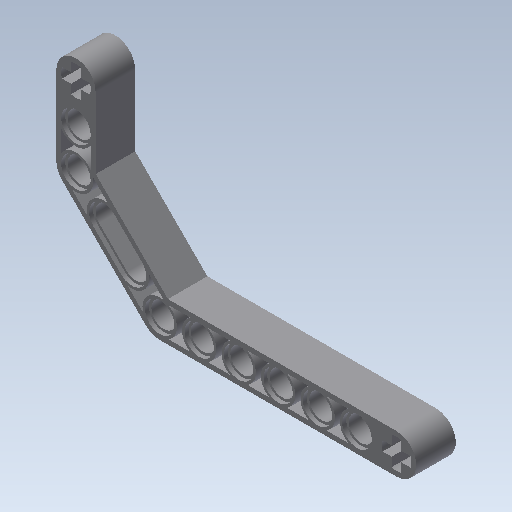
# Autodesk Inventor part: Arm Beam
Saved by Autodesk Inventor 2020 (Build 240168000, 168)
## iProperties
Created: 2014-02-19
Part Number: Arm Beam
Document SubType Name: Modeling
Designer: jleonard
Density: 1 g/cm^3
Material: Generic
Appearance: Default
Author: jleonard
Autodesk Inventor part; units mm, degrees
ref_plane "YZ Plane" through (0, 0, 0) normal (1, 0, 0) x (0, 1, 0)
ref_plane "XZ Plane" through (0, 0, 0) normal (0, 1, 0) x (-1, 0, 0)
ref_plane "XY Plane" through (0, 0, 0) normal (0, 0, 1) x (1, 0, 0)
sketch "Sketch1" plane through (0, 0, 0) normal (0, 0, 1) x (1, 0, 0)
  arc A0 (24, -4) -> (24, 4) centre (24, 0) ccw
  arc A1 (-44.9706, 16.9706) -> (-43.799, 14.1421) centre (-40.9706, 16.9706) ccw
  arc A2 (-36.9706, 32.9706) -> (-44.9706, 32.9706) centre (-40.9706, 32.9706) ccw
  line L0 (24, 4) -> (-22.3431, 4)
  line L1 (-22.3431, 4) -> (-36.9706, 18.6274)
  line L2 (-36.9706, 18.6274) -> (-36.9706, 32.9706)
  line L3 (24, -4) -> (-24, -4)
  line L4 (-26.8284, -2.8284) -> (-43.799, 14.1421)
  line L5 (-44.9706, 16.9706) -> (-44.9706, 32.9706)
  arc A3 (-26.8284, -2.8284) -> (-24, -4) centre (-24, 0) ccw
  line L6 (-59.9022, 0) -> (42.6504, 0) projected
  line L7 (0, -12.5317) -> (0, 45.2209) projected
  point P0 (0, 0)
  dimension "d4" = 48
  dimension "d6" = 16
  dimension "d9" = 24
  dimension "d12" = 4
  dimension "d13" = 4
  dimension "d14" = 4
  dimension "d15" = 4
  dimension "d16" = 135
  dimension "d17" = 135
  dimension "d18" = 4
  dimension "d19" = 4
  dimension "d20" = 4
  dimension "d21" = 4
  dimension "d22" = 24
  dimension "d23" = 0
  dimension "d25" = 4
  dimension "d26" = 4
  dimension "d27" = 8
  dimension "d28" = 8
  dimension "d29" = 22.3432
  dimension "d30" = 36.9706
  constraints: 12 end point, 8 point on circle, 4 centre point, 2 perpendicular
  measures "d4" distance of A3.centre A0.centre
  measures "d6" distance of A1.centre A2.centre
  measures "d9" distance of A3.centre A1.centre
  measures "d12" radius of A2
  measures "d13" radius of A1
  measures "d14" radius of A3
  measures "d15" radius of A0
  measures "d16" angle of L0 L1
  measures "d17" angle of L4 L3
  measures "d18" distance from line of L3 A0.centre
  measures "d19" distance from line of L2 A2.centre
  measures "d20" distance from line of L4 A1.centre
  measures "d21" distance from line of L1 A3.centre
  measures "d22" distance from line of A0.centre L7
  measures "d23" distance from line of A0.centre L6
  measures "d25" distance from line of L1 A1.centre
  measures "d26" distance from line of L0 A3.centre
  measures "d27" distance between parallel lines of L5 L2
  measures "d28" distance between parallel lines of L3 L0
  measures "d29" distance from line of L7 L0.end
  measures "d30" distance from line of L7 L1.end
extrude "Extrusion1" add sketch "Sketch1" along normal blind 8
sketch "Sketch2" plane through (0, 0, 8) normal (0, 0, 1) x (1, 0, 0)
  arc A0 (24, -4) -> (24, 4) centre (24, 0) ccw projected
  line L0 (24, -4) -> (-24, -4) projected
  arc A1 (21.1716, 1) -> (21.1716, -1) centre (24, 0) ccw
  arc A2 (23, -2.8284) -> (25, -2.8284) centre (24, 0) ccw
  arc A3 (26.8284, -1) -> (26.8284, 1) centre (24, 0) ccw
  arc A4 (25, 2.8284) -> (23, 2.8284) centre (24, 0) ccw
  line L1 (21.1716, 1) -> (23, 1)
  line L2 (25, 1) -> (26.8284, 1)
  line L3 (23, -2.8284) -> (23, -1)
  line L4 (23, 1) -> (23, 2.8284)
  line L5 (21.1716, -1) -> (23, -1)
  line L6 (25, -1) -> (26.8284, -1)
  line L7 (25, 2.8284) -> (25, 1)
  line L8 (25, -1) -> (25, -2.8284)
  point P0 (0, 0)
  dimension "d34" = 3
  dimension "d35" = 3
  dimension "d36" = 3
  dimension "d37" = 3
  dimension "d38" = 2
  dimension "d39" = 2
  dimension "d40" = 2
  dimension "d41" = 2
  dimension "d42" = 1
  dimension "d43" = 1
  dimension "d44" = 1
  dimension "d45" = 1
  constraints: 16 end point, 8 parallel, 8 point on circle, 6 perpendicular, 4 centre point, 1 coincident
  measures "d34" radius of A4
  measures "d35" radius of A3
  measures "d36" radius of A2
  measures "d37" radius of A1
  measures "d38" distance between parallel lines of L7 L4
  measures "d39" distance between parallel lines of L5 L1
  measures "d40" distance between parallel lines of L6 L2
  measures "d41" distance between parallel lines of L8 L3
  measures "d42" distance from line of A0.centre L4
  measures "d43" distance from line of A0.centre L1
  measures "d44" distance from line of A0.centre L3
  measures "d45" distance from line of L6 A0.centre
extrude "Extrusion2" cut sketch "Sketch2" against normal through all
sketch "Sketch3" plane through (0, 0, 8) normal (0, 0, 1) x (1, 0, 0)
  arc A0 (-36.9706, 32.9706) -> (-44.9706, 32.9706) centre (-40.9706, 32.9706) ccw projected
  line L0 (24, -4) -> (-24, -4) projected
  arc A1 (-39.9706, 35.799) -> (-41.9706, 35.799) centre (-40.9706, 32.9706) ccw
  arc A2 (-43.799, 33.9706) -> (-43.799, 31.9706) centre (-40.9706, 32.9706) ccw
  arc A3 (-41.9706, 30.1421) -> (-39.9706, 30.1421) centre (-40.9706, 32.9706) ccw
  arc A4 (-38.1421, 31.9706) -> (-38.1421, 33.9706) centre (-40.9706, 32.9706) ccw
  line L1 (-39.9706, 30.1421) -> (-39.9706, 31.9706)
  line L2 (-39.9706, 33.9706) -> (-39.9706, 35.799)
  line L3 (-43.799, 33.9706) -> (-41.9706, 33.9706)
  line L4 (-39.9706, 33.9706) -> (-38.1421, 33.9706)
  line L5 (-41.9706, 30.1421) -> (-41.9706, 31.9706)
  line L6 (-41.9706, 33.9706) -> (-41.9706, 35.799)
  line L7 (-43.799, 31.9706) -> (-41.9706, 31.9706)
  line L8 (-39.9706, 31.9706) -> (-38.1421, 31.9706)
  point P0 (0, 0)
  dimension "d49" = 3
  dimension "d50" = 2
  dimension "d51" = 3
  dimension "d52" = 2
  dimension "d53" = 3
  dimension "d54" = 2
  dimension "d55" = 3
  dimension "d56" = 2
  dimension "d57" = 1
  dimension "d58" = 1
  dimension "d59" = 1
  dimension "d60" = 1
  constraints: 16 end point, 8 parallel, 8 point on circle, 6 perpendicular, 4 centre point, 1 coincident
  measures "d49" radius of A1
  measures "d50" distance between parallel lines of L2 L6
  measures "d51" radius of A4
  measures "d52" distance between parallel lines of L8 L4
  measures "d53" radius of A3
  measures "d54" distance between parallel lines of L5 L1
  measures "d55" radius of A2
  measures "d56" distance between parallel lines of L7 L3
  measures "d57" distance from line of A0.centre L6
  measures "d58" distance from line of L3 A0.centre
  measures "d59" distance from line of L5 A0.centre
  measures "d60" distance from line of L8 A0.centre
extrude "Extrusion3" cut sketch "Sketch3" against normal through all
sketch "Sketch4" plane through (0, 0, 8) normal (0, 0, 1) x (1, 0, 0)
  arc A0 (-26.8284, -2.8284) -> (-24, -4) centre (-24, 0) ccw projected
  circle A1 centre (-24, 0) radius 2.5
  line L0 (-59.9022, 0) -> (42.6504, 0) projected
  circle A2 centre (-16, 0) radius 2.5
  circle A3 centre (-8, 0) radius 2.5
  circle A4 centre (0, 0) radius 2.5
  circle A5 centre (8, 0) radius 2.5
  circle A6 centre (16, 0) radius 2.5
  point P0 (0, 0)
  dimension "d63" = 5
  dimension "d69" = 8
  constraints: 6 centre point, 1 coincident, 1 horizontal, 10 other
  measures "d63" diameter of A1
  measures "d69" distance of A1.centre A2.centre
extrude "Extrusion4" cut sketch "Sketch4" against normal through all
sketch "Sketch5" plane through (0, 0, 8) normal (0, 0, 1) x (1, 0, 0)
  arc A0 (-44.9706, 16.9706) -> (-43.799, 14.1421) centre (-40.9706, 16.9706) ccw projected
  circle A1 centre (-40.9706, 16.9706) radius 2.5
  line L0 (0, -12.5317) -> (0, 45.2209) projected
  circle A2 centre (-40.9706, 24.9706) radius 2.5
  dimension "d74" = 5
  dimension "d80" = 8
  constraints: 2 centre point, 1 coincident, 1 vertical, 2 other
  measures "d74" diameter of A1
  measures "d80" distance of A1.centre A2.centre
extrude "Extrusion5" cut sketch "Sketch5" against normal through all
sketch "Sketch6" plane through (0, 0, 8) normal (0, 0, 1) x (1, 0, 0)
  circle A0 centre (-40.9706, 16.9706) radius 2.5 projected
  circle A1 centre (-24, 0) radius 2.5 projected
  line L0 (-36.9706, 18.6274) -> (-22.3431, 4) projected
  line L1 (-26.8284, -2.8284) -> (-43.799, 14.1421) projected
  arc A2 (-33.5459, 13.0815) -> (-37.0815, 9.5459) centre (-35.3137, 11.3137) ccw
  arc A3 (-31.4246, 3.8891) -> (-27.8891, 7.4246) centre (-29.6569, 5.6569) ccw
  line L2 (-33.5459, 13.0815) -> (-27.8891, 7.4246)
  line L3 (-31.4246, 3.8891) -> (-37.0815, 9.5459)
  dimension "d111" = 2.5
  dimension "d112" = 2.5
  dimension "d115" = 0
  dimension "d116" = 4
  dimension "d117" = 5
  dimension "d118" = 2.5
  dimension "d119" = 8
  dimension "d120" = 8
  constraints: 4 end point, 4 point on circle, 2 centre point, 1 parallel, 1 point on line, 1 tangent
  measures "d111" radius of A2
  measures "d112" radius of A3
  measures "d115" angle of L3 L0
  measures "d116" distance from line of L1 A3.centre
  measures "d117" distance between parallel lines of L2 L3
  measures "d118" distance from line of L3 A2.centre
  measures "d119" distance of A2.centre A0.centre
  measures "d120" distance of A1.centre A3.centre
extrude "Extrusion6" cut sketch "Sketch6" against normal through all contours L2 A3 L3 A2
sketch "Sketch7" plane through (0, 0, 8) normal (0, 0, 1) x (1, 0, 0)
  line L0 (-31.4246, 3.8891) -> (-37.0815, 9.5459) projected
  arc A0 (-33.5459, 13.0815) -> (-37.0815, 9.5459) centre (-35.3137, 11.3137) ccw projected
  line L1 (-33.5459, 13.0815) -> (-27.8891, 7.4246) projected
  arc A1 (-31.4246, 3.8891) -> (-27.8891, 7.4246) centre (-29.6569, 5.6569) ccw projected
  circle A2 centre (-40.9706, 24.9706) radius 2.5 projected
  circle A3 centre (-40.9706, 16.9706) radius 2.5 projected
  circle A4 centre (16, 0) radius 2.5 projected
  circle A5 centre (8, 0) radius 2.5 projected
  circle A6 centre (0, 0) radius 2.5 projected
  circle A7 centre (-8, 0) radius 2.5 projected
  circle A8 centre (-16, 0) radius 2.5 projected
  circle A9 centre (-24, 0) radius 2.5 projected
  arc A10 (-44.9706, 16.9706) -> (-43.799, 14.1421) centre (-40.9706, 16.9706) ccw projected
  arc A11 (-26.8284, -2.8284) -> (-24, -4) centre (-24, 0) ccw projected
  line L2 (-27.5355, 7.7782) -> (-33.1924, 13.435)
  arc A12 (-33.1924, 13.435) -> (-37.435, 9.1924) centre (-35.3137, 11.3137) ccw
  line L3 (-37.435, 9.1924) -> (-31.7782, 3.5355)
  arc A13 (-31.7782, 3.5355) -> (-27.5355, 7.7782) centre (-29.6569, 5.6569) ccw
  circle A14 centre (-40.9706, 24.9706) radius 3
  circle A15 centre (-40.9706, 16.9706) radius 3
  circle A16 centre (-24, 0) radius 3
  circle A17 centre (-16, 0) radius 3
  circle A18 centre (-8, 0) radius 3
  circle A19 centre (0, 0) radius 3
  circle A20 centre (8, 0) radius 3
  circle A21 centre (16, 0) radius 3
  dimension "d123" = 6
  dimension "d124" = 6
  dimension "d125" = 6
  dimension "d126" = 6
  dimension "d127" = 6
  dimension "d128" = 6
  dimension "d129" = 3
  dimension "d130" = 6
  dimension "d131" = 6
  constraints: 10 centre point, 8 coincident, 4 end point, 4 point on circle, 3 other
  measures "d123" diameter of A21
  measures "d124" diameter of A20
  measures "d125" diameter of A19
  measures "d126" diameter of A18
  measures "d127" diameter of A17
  measures "d128" diameter of A16
  measures "d129" radius of A13
  measures "d130" diameter of A15
  measures "d131" diameter of A14
extrude "Extrusion7" cut sketch "Sketch7" against normal blind 0.8
sketch "Sketch8" plane through (0, 0, 0) normal (0, 0, -1) x (-1, 0, 0)
  line L0 (37.0815, 9.5459) -> (31.4246, 3.8891) projected
  arc A0 (27.8891, 7.4246) -> (31.4246, 3.8891) centre (29.6569, 5.6569) ccw projected
  line L1 (27.8891, 7.4246) -> (33.5459, 13.0815) projected
  arc A1 (37.0815, 9.5459) -> (33.5459, 13.0815) centre (35.3137, 11.3137) ccw projected
  circle A2 centre (40.9706, 24.9706) radius 2.5 projected
  circle A3 centre (40.9706, 16.9706) radius 2.5 projected
  circle A4 centre (-16, 0) radius 2.5 projected
  circle A5 centre (-8, 0) radius 2.5 projected
  circle A6 centre (0, 0) radius 2.5 projected
  circle A7 centre (8, 0) radius 2.5 projected
  circle A8 centre (16, 0) radius 2.5 projected
  circle A9 centre (24, 0) radius 2.5 projected
  arc A10 (24, -4) -> (26.8284, -2.8284) centre (24, 0) ccw projected
  arc A11 (43.799, 14.1421) -> (44.9706, 16.9706) centre (40.9706, 16.9706) ccw projected
  circle A12 centre (40.9706, 24.9706) radius 3
  circle A13 centre (40.9706, 16.9706) radius 3
  circle A14 centre (24, 0) radius 3
  circle A15 centre (16, 0) radius 3
  circle A16 centre (8, 0) radius 3
  circle A17 centre (0, 0) radius 3
  circle A18 centre (-8, 0) radius 3
  circle A19 centre (-16, 0) radius 3
  line L2 (31.7782, 3.5355) -> (37.435, 9.1924)
  arc A20 (37.435, 9.1924) -> (33.1924, 13.435) centre (35.3137, 11.3137) ccw
  line L3 (33.1924, 13.435) -> (27.5355, 7.7782)
  arc A21 (27.5355, 7.7782) -> (31.7782, 3.5355) centre (29.6569, 5.6569) ccw
  dimension "d134" = 6
  dimension "d135" = 6
  dimension "d136" = 6
  dimension "d137" = 6
  dimension "d138" = 6
  dimension "d139" = 6
  dimension "d140" = 6
  dimension "d141" = 6
  dimension "d142" = 3
  constraints: 10 centre point, 8 coincident, 4 end point, 4 point on circle, 3 other
  measures "d134" diameter of A19
  measures "d135" diameter of A18
  measures "d136" diameter of A17
  measures "d137" diameter of A16
  measures "d138" diameter of A15
  measures "d139" diameter of A14
  measures "d140" diameter of A13
  measures "d141" diameter of A12
  measures "d142" radius of A20
extrude "Extrusion8" cut sketch "Sketch8" against normal blind 0.8
sketch "Sketch9" plane through (0, 0, 8) normal (0, 0, 1) x (1, 0, 0)
  circle A0 centre (-40.9706, 24.9706) radius 3 projected
  circle A1 centre (-40.9706, 16.9706) radius 3 projected
  circle A2 centre (-24, 0) radius 3 projected
  circle A3 centre (-16, 0) radius 3 projected
  circle A4 centre (-8, 0) radius 3 projected
  circle A5 centre (0, 0) radius 3 projected
  circle A6 centre (8, 0) radius 3 projected
  circle A7 centre (16, 0) radius 3 projected
  arc A8 (-33.1924, 13.435) -> (-37.435, 9.1924) centre (-35.3137, 11.3137) ccw projected
  arc A9 (-31.7782, 3.5355) -> (-27.5355, 7.7782) centre (-29.6569, 5.6569) ccw projected
  arc A10 (-44.9706, 16.9706) -> (-43.799, 14.1421) centre (-40.9706, 16.9706) ccw projected
  line L0 (-26.8284, -2.8284) -> (-43.799, 14.1421) projected
  arc A11 (-26.8284, -2.8284) -> (-24, -4) centre (-24, 0) ccw projected
  line L1 (24, -4) -> (-24, -4) projected
  arc A12 (-22.1972, -3) -> (-22.1972, 3) centre (-24, 0) ccw
  arc A13 (-30.5034, 2.2608) -> (-26.2608, 6.5034) centre (-29.6569, 5.6569) ccw
  arc A14 (-34.4671, 14.7098) -> (-38.7098, 10.4671) centre (-35.3137, 11.3137) ccw
  arc A15 (-43.9706, 23.1678) -> (-37.9714, 23.1664) centre (-40.9706, 24.9706) ccw
  arc A16 (14.1972, 3) -> (14.1972, -3) centre (16, 0) ccw
  line L2 (9.8028, 3) -> (14.1972, 3)
  line L3 (9.8028, -3) -> (14.1972, -3)
  line L4 (-22.1972, -3) -> (-17.8028, -3)
  line L5 (-14.1972, -3) -> (-9.8028, -3)
  line L6 (-6.1972, -3) -> (-1.8028, -3)
  line L7 (1.8028, -3) -> (6.1972, -3)
  line L8 (6.1972, 3) -> (1.8028, 3)
  line L9 (-1.8028, 3) -> (-6.1972, 3)
  line L10 (-9.8028, 3) -> (-14.1972, 3)
  line L11 (-22.1972, 3) -> (-17.8028, 3)
  arc A17 (6.1972, 3) -> (6.1972, -3) centre (8, 0) ccw
  arc A18 (9.8028, -3) -> (9.8028, 3) centre (8, 0) ccw
  arc A19 (1.8028, -3) -> (1.8028, 3) centre (0, 0) ccw
  arc A20 (-1.8028, 3) -> (-1.8028, -3) centre (0, 0) ccw
  arc A21 (-9.8028, 3) -> (-9.8028, -3) centre (-8, 0) ccw
  arc A22 (-6.1972, -3) -> (-6.1972, 3) centre (-8, 0) ccw
  arc A23 (-14.1972, -3) -> (-14.1972, 3) centre (-16, 0) ccw
  arc A24 (-17.8028, 3) -> (-17.8028, -3) centre (-16, 0) ccw
  line L12 (-26.2608, 6.5034) -> (-23.1534, 3.3961)
  line L13 (-30.5034, 2.2608) -> (-27.3961, -0.8466)
  arc A25 (-23.1534, 3.3961) -> (-27.3961, -0.8466) centre (-24, 0) ccw
  line L14 (-38.7098, 10.4671) -> (-41.8171, 13.5745)
  line L15 (-34.4671, 14.7098) -> (-37.5745, 17.8171)
  line L16 (-43.9706, 18.7733) -> (-43.9706, 23.1678)
  arc A26 (-37.9714, 18.7747) -> (-43.9706, 18.7733) centre (-40.9706, 16.9706) ccw
  arc A27 (-41.8171, 13.5745) -> (-37.5745, 17.8171) centre (-40.9706, 16.9706) ccw
  line L17 (-37.9714, 18.7747) -> (-37.9714, 23.1664)
  dimension "d145" = 7
  dimension "d151" = 3.5
  dimension "d152" = 3.5
  dimension "d153" = 3.5
  dimension "d154" = 3.5
  dimension "d155" = 4.3944
  dimension "d156" = 3.5
  dimension "d157" = 3.5
  dimension "d158" = 3.5
  dimension "d159" = 3.5
  dimension "d160" = 3.5
  dimension "d161" = 7
  dimension "d163" = 7
  dimension "d165" = 7
  dimension "d166" = 3.5
  dimension "d167" = 3.5
  dimension "d168" = 3.5
  dimension "d169" = 4.3918
  constraints: 32 end point, 32 point on circle, 20 tangent, 16 centre point, 11 coincident, 6 parallel, 5 collinear, 1 perpendicular
  measures "d145" diameter of A16
  measures "d151" radius of A17
  measures "d152" radius of A18
  measures "d153" radius of A24
  measures "d154" radius of A12
  measures "d155" distance of L4.start L4.end
  measures "d156" radius of A23
  measures "d157" radius of A21
  measures "d158" radius of A22
  measures "d159" radius of A20
  measures "d160" radius of A19
  measures "d161" diameter of A13
  measures "d163" diameter of A14
  measures "d165" diameter of A15
  measures "d166" radius of A25
  measures "d167" radius of A27
  measures "d168" radius of A26
  measures "d169" distance of L17.start L17.end
extrude "Extrusion9" cut sketch "Sketch9" against normal through all contours A12 L11 A24 L4 | A13 L12 A25 L13 | A14 L14 A27 L15 | A15 L17 A26 L16 | A16 L3 A18 L2 | A23 L10 A21 L5 | A22 L9 A20 L6 | A19 L8 A17 L7
body "Solid1"
